Autodesk Fusion 360 part; units mm, degrees
note: some values were not read from the file. Chosen so that the rebuilt part matches the saved one: that a step has no effect.
(part 3 of 3)
  spline S170 degree 3 poles (-104.2491, 17.2744) (-104.3409, 17.035) (-104.0197, 16.9576) (-103.8031, 17.1643) knots 0 0 0 0 1 1 1 1
  spline S171 degree 3 poles (-103.8031, 17.1643) (-103.6335, 17.3281) (-103.6498, 17.3649) (-103.9014, 17.3852) knots 0 0 0 0 1 1 1 1
  spline S172 degree 3 poles (-104.0882, 15.626) (-105.0474, 15.5515) (-105.0842, 15.5351) (-104.8547, 15.0199) knots 0 0 0 0 1 1 1 1
  spline S173 degree 3 poles (-104.8547, 15.0199) (-104.658, 14.5782) (-104.2652, 14.4886) (-103.6395, 14.7673) knots 0 0 0 0 1 1 1 1
  spline S174 degree 3 poles (-103.6395, 14.7673) (-103.3819, 14.882) (-103.235, 15.3444) (-103.3661, 15.6388) knots 0 0 0 0 1 1 1 1
  spline S175 degree 3 poles (-103.3661, 15.6388) (-103.3743, 15.6572) (-103.6996, 15.6447) (-104.0882, 15.626) knots 0 0 0 0 1 1 1 1
  spline S176 degree 3 poles (-103.6881, 11.6582) (-104.0377, 11.5025) (-104.0434, 10.9707) (-103.7016, 10.748) knots 0 0 0 0 1 1 1 1
  spline S177 degree 3 poles (-103.7016, 10.748) (-103.5358, 10.6234) (-103.4418, 10.7094) (-103.3644, 11.0306) knots 0 0 0 0 1 1 1 1
  spline S178 degree 3 poles (-103.3644, 11.0306) (-103.2483, 11.6115) (-103.3384, 11.814) (-103.6881, 11.6582) knots 0 0 0 0 1 1 1 1
extrude "Extrusion13" cut sketch "Esquisse24" against normal blind 1.5 contours S0 S1 L8 L9 S2 S3 S4 S5 S6 S7 S8 S9 S10 S11 | S12 S13 S14 S15 S16 S17 S18 S19 | S20 S21 S22 S23 S24 S25 S26 S27 S28 | S29 S30 S31 S32 S33 S34 S35 S36 S37 S38 S39 S40 S41 S42 S43 S44 S45 S46 S47 S48 S49 S50 S51 S52 S53 S54 S55 S56 S57 | S58 S59 L10 L11 S60 S61 S62 | S63 S64 S65 S66 S67 S68 S69 S70 | S71 S72 S73 | S74 S75 S76 S77 S78 | S79 S80 S81 S82 S83 S84 S85 | S86 S87 S88 S89 S90 | S91 S92 S93 S94 L12 L13 L14 L15 S95 S96 S97 | S98 S99 S100 S101 | S102 S103 S104 S105 S106 S107 S108 S109 S110 S111 | S112 S113 S114 S115 S116 S117 S118 S119 S120 S121 S122 S123 S124 | S125 S126 L16 L17 S127 S128 | S129 S130 S131 S132 | S133 S134 S135 S136 S137 S138 S139 S140 S141 L18 L19 S142 | S143 S144 S145 S146 S147 S148 S149 S150 bodies 4 in component "Component'"
extrude "Extrusion14" cut 1 faces at (77.1406, 66.4502, 138.3107) along direction (0, 0, 1) blind 1 on bodies 4 bodies 4 in component "Component'"
extrude "Extrusion15" cut 1 faces at (43.0473, 66.4502, -0.4393) along direction (0, 0, -1) blind 1 on bodies 4 bodies 4 in component "Component'"
extrude "Extrusion16" cut 1 faces at (8.9539, 69.7835, 92.3941) along direction (-1, 0, 0) blind 0.735 on bodies 4 bodies 4 in component "Component'"
extrude "Extrusion17" cut 1 faces at (111.2339, 66.4502, 45.4774) along direction (1, 0, 0) blind 0.735 on bodies 4 bodies 4 in component "Component'"
extrude "Extrusion18" cut 1 faces at (77.3856, 69.7835, -1.4393) along direction (0, 0, -1) blind 0.5 on bodies 4 bodies 4 in component "Component'"
extrude "Extrusion19" cut 1 faces at (77.3856, 69.7835, 139.3107) along direction (0, 0, 1) blind 0.5 on bodies 4 bodies 4 in component "Component'"
component "Component" placed x (1, 0, 0) y (0, 1, 0) z (0, 0, 1) at (0, 0, 0)
component "Component'" placed x (1, 0, 0) y (0, 1, 0) z (0, 0, 1) at (0, 0, 0)
